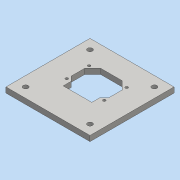
# Autodesk Inventor part: Camera-Holder_Mount
Saved by Autodesk Inventor 2016 SP1 (Build 200210100, 210)
## iProperties
Created: 2016-02-08
Part Number: Camera-Holder_Mount
Material: Generic
Document SubType Name: Modeling
Designer: Mohamed A.
Density: 1 g/cm^3
Appearance: Default
Author: Mohamed A.
Autodesk Inventor part; units mm, degrees
ref_plane "YZ Plane" through (0, 0, 0) normal (1, 0, 0) x (0, 1, 0)
ref_plane "XZ Plane" through (0, 0, 0) normal (0, 1, 0) x (-1, 0, 0)
ref_plane "XY Plane" through (0, 0, 0) normal (0, 0, 1) x (1, 0, 0)
sketch "Sketch1" plane through (0, 0, 0) normal (0, 0, 1) x (1, 0, 0)
  circle A0 centre (-10.5, 10) radius 0.75
  circle A1 centre (-10.5, -2.5) radius 0.75
  circle A2 centre (10.5, 10) radius 0.75
  circle A3 centre (10.5, -2.5) radius 0.75
  line L0 (6, 12) -> (10.5, 7.5)
  line L1 (10.5, 7.5) -> (10.5, 0)
  line L2 (0, 15.2771) -> (0, -20.9272) construction
  line L3 (10.5, 0) -> (8, -2.5)
  line L4 (8, -2.5) -> (8, -7)
  line L5 (-6, 12) -> (-10.5, 7.5)
  line L6 (-10.5, 7.5) -> (-10.5, 0)
  line L7 (-10.5, 0) -> (-8, -2.5)
  line L8 (-8, -2.5) -> (-8, -7)
  line L9 (8, -7) -> (-8, -7)
  line L10 (23.5, 23.5) -> (23.5, -23.5)
  line L11 (23.5, -23.5) -> (-23.5, -23.5)
  line L12 (-23.5, -23.5) -> (-23.5, 23.5)
  line L13 (-23.5, 23.5) -> (23.5, 23.5)
  line L14 (6, 12) -> (-6, 12)
  line L15 (12.5, 12.5) -> (12.5, -12.5) construction
  line L16 (-12.5, -12.5) -> (-12.5, 12.5) construction
  line L17 (12.5, -12.5) -> (23.5, -23.5) construction
  line L18 (12.5, 12.5) -> (23.5, 23.5) construction
  line L19 (-12.5, 12.5) -> (-23.5, 23.5) construction
  line L20 (-12.5, -12.5) -> (-23.5, -23.5) construction
  circle A4 centre (18, -18) radius 1.4
  circle A5 centre (18, 18) radius 1.4
  circle A6 centre (-18, 18) radius 1.4
  circle A7 centre (-18, -18) radius 1.4
  line L21 (12.5, 12.5) -> (-12.5, -12.5) construction
  line L22 (12.5, -12.5) -> (-12.5, 12.5) construction
  point P0 (0, 0)
  point P1 (0, 0)
  point P2 (0, 0)
  point P3 (-8.25, 9.75)
  point P4 (0, 0)
  point P5 (0, 0)
  dimension "d2" = 1.5
  dimension "d5" = 1.5
  dimension "d8" = 1.5
  dimension "d11" = 1.5
  dimension "d48" = 2.8
  dimension "d49" = 2.8
  dimension "d50" = 2.8
  dimension "d51" = 2.8
  dimension "d63" = 15.5564
  dimension "d64" = 7.7782
  dimension "d66" = 7.7782
  dimension "d67" = 7.7782
  dimension "d68" = 47
  constraints: 46 end point, 9 vertical, 8 centre point, 8 midpoint, 5 perpendicular, 4 symmetric about line, 3 collinear, 3 horizontal, 1 coincident, 1 point on line, 9 other
  measures "d2" diameter of A0
  measures "d5" diameter of A1
  measures "d8" diameter of A2
  measures "d11" diameter of A3
  measures "d48" diameter of A4
  measures "d49" diameter of A5
  measures "d50" diameter of A6
  measures "d51" diameter of A7
  measures "d63" distance of L15.start L10.start
  measures "d64" distance of L15.start A5.centre
  measures "d66" distance of A6.centre L16.end
  measures "d67" distance of L16.start A7.centre
  measures "d68" distance between parallel lines of L12 L10
extrude "Extrusion1" add sketch "Sketch1" along normal blind 3
equation "\"d64\" = 0.5 * d63"
equation "\"d66\" = d64"
equation "\"d67\" = d64"
body "Solid1"
